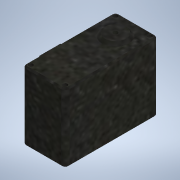
# Autodesk Inventor part: motor_body
Saved by Autodesk Inventor 2020 (Build 240168000, 168)
## iProperties
Created: 2020-08-28
Part Number: motor_body
Material: 일반
Document SubType Name: Modeling
Designer: qwer1
Density: 1 g/cm^3
Appearance: 매끄러움 - 검은색
Author: qwer1
Autodesk Inventor part; units mm, degrees
ref_plane "YZ Plane" through (0, 0, 0) normal (1, 0, 0) x (0, 1, 0)
ref_plane "XZ Plane" through (0, 0, 0) normal (0, 1, 0) x (-1, 0, 0)
ref_plane "XY Plane" through (0, 0, 0) normal (0, 0, 1) x (1, 0, 0)
sketch "스케치1" plane through (0, 0, 0) normal (0, 1, 0) x (-1, 0, 0)
  line L0 (-3, 0) -> (-27, 0)
  line L1 (-30, -3) -> (-30, -62)
  line L2 (-27, -65) -> (-3, -65)
  line L3 (0, -62) -> (0, -3)
  arc A0 (-3, -65) -> (0, -62) centre (-3, -62) ccw
  arc A1 (-30, -62) -> (-27, -65) centre (-27, -62) ccw
  arc A2 (0, -3) -> (-3, 0) centre (-3, -3) ccw
  arc A3 (-27, 0) -> (-30, -3) centre (-27, -3) ccw
  circle A4 centre (-15, -50) radius 9.285
  circle A5 centre (-27, -62) radius 3
  circle A6 centre (-27, -62) radius 1.25
  circle A7 centre (-3, -62) radius 3
  circle A8 centre (-3, -62) radius 1.25
  circle A9 centre (-3, -3) radius 3
  circle A10 centre (-3, -3) radius 1.25
  circle A11 centre (-27, -3) radius 3
  circle A12 centre (-27, -3) radius 1.25
  circle A13 centre (-27, -62) radius 3
  circle A14 centre (-27, -62) radius 1.25
  point P0 (0, 0)
  point P1 (-2.9832, -51.69)
  dimension "d2" = 3
  dimension "d21" = 2.5
  dimension "d22" = 2.5
  dimension "d23" = 2.5
  dimension "d24" = 2.5
  dimension "d25" = 2.5
  constraints: 15 centre point, 8 end point, 8 point on circle, 8 tangent, 6 coincident, 3 equal radius, 2 parallel, 2 point on line, 1 horizontal, 1 perpendicular
  measures "d2" radius of A0
  measures "d21" diameter of A6
  measures "d22" diameter of A8
  measures "d23" diameter of A10
  measures "d24" diameter of A12
  measures "d25" diameter of A14
extrude "돌출1" add sketch "스케치1" along normal blind 48 contours A9 L3 A7 L2 A5 L1 A11 L0 | A2 A9 | A11 A3 | A0 A7 | A5 A1 | A4 | A6 | A8 | A10 | A12
extrude "돌출2" add sketch "스케치1" against normal blind 2 contours A4
extrude "돌출3" add sketch "스케치1" along normal blind 50 contours A4
chamfer "모따기1" distance 2 angle 45 1 edges at (24.285, -2, -50)
chamfer "모따기2" distance 2 angle 45 1 edges at (24.285, 50, -50)
sketch "스케치2" plane through (15, -2, -50) normal (0, -1, 0) x (1, 0, 0)
  circle A0 centre (0, 0) radius 1.5
  point P0 (-15, 50)
  dimension "d15" = 3
  constraints: 1 centre point
  measures "d15" diameter of A0
extrude "돌출4" cut sketch "스케치2" against normal blind 52
chamfer "모따기3" distance 1 angle 45 16 edges at (15, 0, -65) (0.8787, 0, -64.1213) (0, 0, -32.5) (0.8787, 0, -0.8787) (15, 0, 0) (29.1213, 0, -0.8787) (30, 0, -32.5) (29.1213, 0, -64.1213) (0.8787, 48, -64.1213) (0, 48, -32.5) (0.8787, 48, -0.8787) (15, 48, 0) (29.1213, 48, -0.8787) (30, 48, -32.5) (29.1213, 48, -64.1213) (15, 48, -65)
sketch "스케치3" plane through (0, 48, 0) normal (0, 1, 0) x (1, 0, 0)
  circle A0 centre (27, 62) radius 1.25 projected
  circle A1 centre (3, 62) radius 1.25 projected
  circle A2 centre (27, 3) radius 1.25 projected
  circle A3 centre (3, 3) radius 1.25 projected
  circle A4 centre (15, 50) radius 9.285 projected
  arc A5 (3, 64) -> (1, 62) centre (3, 62) ccw projected
  line L0 (1, 3) -> (1, 62) projected
  arc A6 (1, 3) -> (3, 1) centre (3, 3) ccw projected
  line L1 (27, 1) -> (3, 1) projected
  arc A7 (27, 1) -> (29, 3) centre (27, 3) ccw projected
  line L2 (29, 62) -> (29, 3) projected
  arc A8 (29, 62) -> (27, 64) centre (27, 62) ccw projected
  line L3 (3, 64) -> (27, 64) projected
  point P0 (0, 0)
hole "구멍1" at (27, 0, -62) at (3, 0, -62) at (3, 0, -3) at (27, 0, -3) direction (0, 1, 0) diameter 3 depth 10 tip angle 118
hole "구멍2" at (3, 48, -62) at (27, 48, -62) at (27, 48, -3) at (3, 48, -3) direction (0, -1, 0) diameter 3 depth 10 tip angle 118
sketch "스케치4" plane through (0, 1, -62) normal (-1, 0, 0) x (0, 0, 1)
  line L0 (0, 0) -> (59, 0) projected
  line L1 (59, 46) -> (0, 46) projected
  line L2 (34.8314, 0) -> (49.601, 0)
  line L3 (49.601, 0) -> (49.601, 46)
  line L4 (49.601, 46) -> (34.8314, 46)
  line L5 (34.8314, 46) -> (34.8314, 0)
  line L6 (42.3157, -29.4705) -> (42.3157, -13.5566) construction
  line L7 (42.3157, -13.5566) -> (78.2048, -13.5566) construction
  line L8 (78.2048, -13.5566) -> (78.2048, -29.4705) construction
  line L9 (78.2048, -29.4705) -> (42.3157, -29.4705) construction
  point P0 (62, -1)
  constraints: 8 end point, 2 parallel, 2 point on line, 1 horizontal, 1 perpendicular, 2 other
extrude "돌출5" add sketch "스케치4" along normal blind 0.5
sketch "스케치5" plane through (-0.5, 1, -62) normal (-1, 0, 0) x (0, 0, 1)
  line L0 (40.8953, 14.0601) -> (40.786, 33.6253) construction
  line L1 (40.786, 33.6253) -> (43.962, 33.643) construction
  line L2 (43.962, 33.643) -> (44.0713, 14.0778) construction
  line L3 (44.0713, 14.0778) -> (40.8953, 14.0601) construction
  constraints: 2 other
